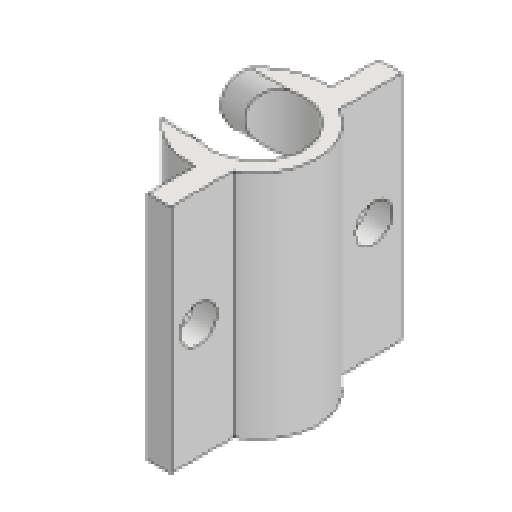
# Autodesk Inventor part: LinearClampPart2
Saved by Autodesk Inventor 2023 (Build 270158000, 158)
## iProperties
Created: 2022-10-30
Part Number: LinearClampPart2
Material: Generic
Document SubType Name: Modeling
Designer: deli
Density: 1 g/cm^3
Appearance: Default
Author: deli
Autodesk Inventor part; units mm, degrees
ref_plane "YZ Plane" through (0, 0, 0) normal (1, 0, 0) x (0, 1, 0)
ref_plane "XZ Plane" through (0, 0, 0) normal (0, 1, 0) x (-1, 0, 0)
ref_plane "XY Plane" through (0, 0, 0) normal (0, 0, 1) x (1, 0, 0)
sketch "Sketch1" plane through (0, 0, 0) normal (0, 1, 0) x (-1, 0, 0)
  circle A0 centre (12.5275, -32.6585) radius 4
  line L0 (12.0275, -42.6585) -> (10.0275, -42.6585)
  line L1 (10.0275, -22.6585) -> (12.0275, -22.6585)
  line L2 (12.0275, -38.5337) -> (12.0275, -42.6585)
  line L3 (12.0275, -22.6585) -> (12.0275, -26.7833)
  line L4 (10.0275, -28.0818) -> (10.0275, -22.6585)
  line L5 (10.0275, -42.6585) -> (10.0275, -37.2353)
  arc A1 (10.0275, -28.0818) -> (10.0275, -37.2353) centre (12.5275, -32.6585) ccw
  arc A2 (12.0275, -38.5337) -> (12.0275, -26.7833) centre (12.5275, -32.6585) ccw
  point P0 (0, 0)
  dimension "d6" = 8
  dimension "d8" = 20
  dimension "d9" = 0.5
  dimension "d32" = 2
  constraints: 12 end point, 6 perpendicular, 4 point on circle, 3 centre point, 2 equal length, 2 vertical, 1 coincident, 1 collinear
  measures "d6" diameter of A0
  measures "d8" distance between parallel lines of L0 L1
  measures "d9" distance from line of A0.centre L3
  measures "d32" distance between parallel lines of L3 L4
extrude "Extrusion1" add sketch "Sketch1" along normal blind 20
sketch "Sketch3" plane through (-12.0275, 0, -42.6585) normal (-1, 0, 0) x (0, 0, 1)
  circle A0 centre (5, 17.5) radius 2.75
  circle A1 centre (15, 17.5) radius 2.75
  circle A2 centre (5, 2.5) radius 2.75
  circle A3 centre (15, 2.5) radius 2.75
  line L0 (0, 0) -> (4.1248, 0) projected
  line L1 (0, 0) -> (0, 20) projected
  line L2 (0, 20) -> (4.1248, 20) projected
  line L3 (20, 0) -> (20, 20) projected
  line L4 (15.8752, 0) -> (20, 0) projected
  line L5 (15.8752, 20) -> (20, 20) projected
  line L6 (0, 20) -> (20, 20)
  line L7 (20, 20) -> (20, 0)
  line L8 (20, 0) -> (0, 0)
  line L9 (0, 0) -> (0, 20)
  point P0 (42.6585, 0)
  point P1 (6.1456, 0)
  point P2 (13.8544, 0)
  point P3 (16.1456, 0)
  point P4 (16.1456, 20)
  point P5 (13.8544, 20)
  point P6 (6.1456, 20)
  point P7 (3.8544, 20)
  point P8 (3.8544, 0)
  dimension "d23" = 5.5
  dimension "d24" = 2.5
  dimension "d25" = 5
  dimension "d26" = 5
  dimension "d27" = 2.5
  dimension "d28" = 5
  dimension "d29" = 2.5
  dimension "d30" = 2.5
  dimension "d31" = 5
  constraints: 8 end point, 4 centre point, 3 equal radius, 2 parallel, 1 horizontal, 1 perpendicular
  measures "d23" diameter of A0
  measures "d24" distance from line of L0 A2.centre
  measures "d25" distance from line of L1 A2.centre
  measures "d26" distance from line of L1 A0.centre
  measures "d27" distance from line of L2 A0.centre
  measures "d28" distance from line of L3 A3.centre
  measures "d29" distance from line of A3.centre L4
  measures "d30" distance from line of L5 A1.centre
  measures "d31" distance from line of L3 A1.centre
extrude "Extrusion3" cut sketch "Sketch3" along normal blind 6.5 contours A0 L6 A1 L5 L3 L4 A3 L8 A2 L0 L1 L2
sketch "Sketch4" plane through (-10.0275, 0, -22.6585) normal (1, 0, 0) x (0, 0, -1)
  circle A0 centre (2.4, 10) radius 1.6
  circle A1 centre (17.6, 10) radius 1.6
  line L0 (5.4233, 0) -> (5.4233, 20) projected
  line L1 (0, 0) -> (0, 20) projected
  line L2 (0, 20) -> (5.4233, 20) projected
  line L3 (14.5767, 20) -> (20, 20) projected
  line L4 (14.5767, 0) -> (14.5767, 20) projected
  line L5 (20, 0) -> (20, 20) projected
  point P0 (-22.6585, 0)
  dimension "d35" = 3.2
  dimension "d37" = 20
  dimension "d38" = 10
  dimension "d40" = 10
  dimension "d44" = 2.4
  dimension "d45" = 2.4
  constraints: 2 centre point, 1 equal radius
  measures "d35" diameter of A0
  measures "d37" distance of L1.start L1.end
  measures "d38" distance from line of L2 A0.centre
  measures "d40" distance from line of L3 A1.centre
  measures "d44" distance from line of L1 A0.centre
  measures "d45" distance from line of L5 A1.centre
extrude "Extrusion4" cut sketch "Sketch4" against normal blind 10
ref_plane "Work Plane2" through (-16.0275, 0, -42.6585) normal (-1, 0, 0) x (0, 0, 1)
sketch "Sketch5" plane through (-16.0275, 0, -42.6585) normal (-1, 0, 0) x (0, 0, 1)
  line L0 (-6.5958, 31.6476) -> (37.5707, 31.6476)
  line L1 (37.5707, 31.6476) -> (37.5707, -11.0589)
  line L2 (37.5707, -11.0589) -> (-6.5958, -11.0589)
  line L3 (-6.5958, -11.0589) -> (-6.5958, 31.6476)
  point P0 (42.6585, 0)
  constraints: 8 end point, 2 parallel, 1 horizontal, 1 perpendicular
extrude "Extrusion5" cut sketch "Sketch5" along normal blind 10
equation "\"d26\" = d25"
equation "\"d27\" = d24"
equation "\"d28\" = d25"
equation "\"d29\" = d27"
equation "\"d30\" = d27"
equation "\"d31\" = d26"
equation "\"d38\" = 0.5 * d37"
equation "\"d40\" = d38"
equation "\"d45\" = d44"
body "Solid1"
